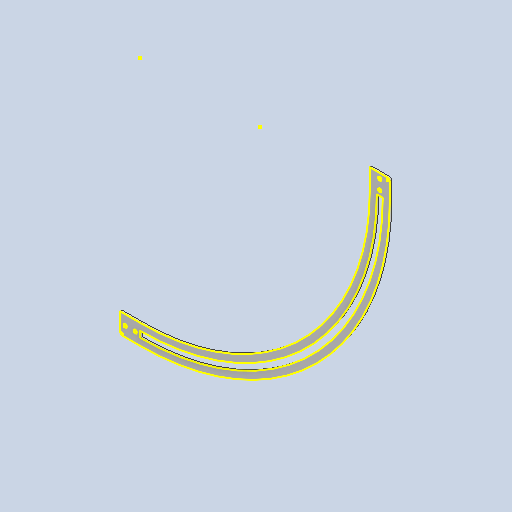
# Autodesk Inventor part: xx_memo
Saved by Autodesk Inventor 2025.1 (Build 291241000, 241)
## iProperties
Created: 2024-12-06
Part Number: xx_memo
Material: 一般
Document SubType Name: Modeling
Designer: yuki0520
Density: 1 g/cm^3
Appearance: 既定
Author: yuki0520
Autodesk Inventor part; units mm, degrees
ref_plane "YZ Plane" through (0, 0, 0) normal (1, 0, 0) x (0, 1, 0)
ref_plane "XZ Plane" through (0, 0, 0) normal (0, 1, 0) x (-1, 0, 0)
ref_plane "XY Plane" through (0, 0, 0) normal (0, 0, 1) x (1, 0, 0)
sketch "スケッチ1" plane through (0, 0, 0) normal (0, 0, 1) x (1, 0, 0)
  line L0 (120, -35) -> (-120, -35)
  line L1 (-120, -35) -> (-120, 35)
  line L2 (-120, 35) -> (120, 35)
  line L3 (120, 35) -> (120, -35)
  line L4 (120, -35) -> (-120, 35) construction
  line L5 (-120, -35) -> (120, 35) construction
  line L6 (-110, -35) -> (-130, -35)
  line L7 (-130, -35) -> (-130, 75)
  line L8 (-130, 75) -> (-110, 75)
  line L9 (-110, 75) -> (-110, -35)
  line L10 (110, 35) -> (130, 35)
  circle A0 centre (-120, 0) radius 6
  line L11 (110, 35) -> (130, 35)
  arc A1 (-120, -240) -> (120, 0) centre (-120, 0) ccw
  arc A2 (-120, -250) -> (130, 0) centre (-120, 0) ccw
  arc A3 (-120, -230) -> (110, 0) centre (-120, 0) ccw
  line L12 (110, 0) -> (130, 0)
  line L13 (130, 0) -> (130, 20)
  line L14 (130, 20) -> (110, 20)
  line L15 (110, 20) -> (110, 0)
  line L16 (-120, -250) -> (-140, -250)
  line L17 (-140, -250) -> (-140, -230)
  line L18 (-140, -230) -> (-120, -230)
  line L19 (-120, -230) -> (-120, -250)
  arc A4 (-120, -243) -> (123, 0) centre (-120, 0) ccw
  arc A5 (-120, -237) -> (117, 0) centre (-120, 0) ccw
  line L20 (130, 20) -> (-140, 20)
  line L21 (-140, 20) -> (-140, -250)
  line L22 (-140, -250) -> (130, -250)
  line L23 (130, -250) -> (130, 20)
  line L24 (-120, -250) -> (-120, 0)
  line L25 (-120, 0) -> (130, 0)
  point P0 (0, 0)
  point P1 (120, 25)
  point P2 (117, 0)
  point P3 (123, 0)
  point P4 (-120, -243)
  point P5 (-120, -237)
  dimension "d0" = 240
  dimension "d1" = 70
  dimension "d2" = 20
  dimension "d3" = 110
  dimension "d4" = 10
  dimension "d8" = 12
  dimension "d14" = 10
  dimension "d18" = 10
  dimension "d19" = 10
  dimension "d20" = 20
  dimension "d21" = 20
  dimension "d22" = 20
  dimension "d23" = 20
  dimension "d26" = 3
  dimension "d27" = 3
  dimension "d37" = 20
  constraints: 52 end point, 10 parallel, 10 point on circle, 7 horizontal, 6 centre point, 6 perpendicular, 4 midpoint, 3 point on line, 1 coincident, 1 other
  measures "d0" distance of L1.end L2.end
  measures "d1" distance of L0.end L1.end
  measures "d2" distance of L7.end L8.end
  measures "d3" distance of L6.end L7.end
  measures "d4" distance between parallel lines of L9 L1
  measures "d8" diameter of A0
  measures "d14" distance from line of L11 point (120, 25)
  measures "d18" radial gap between concentric circles of A1 A2
  measures "d19" radial gap between concentric circles of A1 A3
  measures "d20" distance of L14.end L13.end
  measures "d21" distance of L13.end L12.end
  measures "d22" distance of L18.end L17.end
  measures "d23" distance of L16.end L17.end
  measures "d26" radial gap between concentric circles of A1 A4
  measures "d27" radial gap between concentric circles of A1 A5
  measures "d37" distance between parallel lines of L21 L24
extrude "押し出し1" add sketch "スケッチ1" along normal blind 2 contours A3 L12 A5 L0 | L0 A5 L19 A3 | L19 L16 L17 L18 | L15 L14 L3 L12 | L3 L14 L13 L12 | L19 A4 L12 A2
sketch "スケッチ2" plane through (0, 0, 2) normal (0, 0, 1) x (1, 0, 0)
  line L0 (130, 20) -> (110, 20) projected
  line L1 (120, 20) -> (120, 0)
  line L2 (117, 0) -> (123, 0) projected
  line L3 (-140, -230) -> (-140, -250) projected
  line L4 (-140, -240) -> (-120, -240)
  point P0 (0, 0)
  point P1 (120, 15)
  point P2 (120, 5)
  point P3 (-135, -240)
  point P4 (-125, -240)
  dimension "d28" = 10
  dimension "d29" = 5
  dimension "d52" = 10
  dimension "d53" = 5
  constraints: 4 end point, 4 point on line, 3 midpoint, 1 horizontal
  measures "d28" distance of point (120, 15) point (120, 5)
  measures "d29" distance from line of L0 point (120, 15)
  measures "d52" distance of point (-135, -240) point (-125, -240)
  measures "d53" horizontal distance of L3.start point (-135, -240)
hole "穴1" at (120, 15, 2) at (120, 5, 2) at (-125, -240, 2) at (-135, -240, 2) direction (0, 0, -1) diameter 3.4 end through all
fillet "フィレット1" radius 2 2 edges at (130, 20, 1) (-140, -250, 1)
sketch "スケッチ5" plane through (0, 0, 2) normal (0, 0, 1) x (1, 0, 0)
  arc A0 (-140, -248) -> (-138, -250) centre (-138, -248) ccw projected
  line L0 (-138, -250) -> (-120, -250) projected
  arc A1 (-120, -250) -> (130, 0) centre (-120, 0) ccw projected
  line L1 (130, 0) -> (130, 18) projected
  arc A2 (130, 18) -> (128, 20) centre (128, 18) ccw projected
  line L2 (128, 20) -> (110, 20) projected
  line L3 (110, 20) -> (110, 0) projected
  arc A3 (-120, -230) -> (110, 0) centre (-120, 0) ccw projected
  line L4 (-120, -230) -> (-140, -230) projected
  line L5 (-140, -230) -> (-140, -248) projected
  circle A4 centre (-135, -240) radius 1.7 projected
  circle A5 centre (-125, -240) radius 1.7 projected
  circle A6 centre (120, 5) radius 1.7 projected
  circle A7 centre (120, 15) radius 1.7 projected
  line L6 (117, 0) -> (123, 0) projected
  arc A8 (-120, -243) -> (123, 0) centre (-120, 0) ccw projected
  line L7 (-120, -243) -> (-120, -237) projected
  arc A9 (-120, -237) -> (117, 0) centre (-120, 0) ccw projected
  point P0 (0, 0)
equation "\"d4\" = 0.5 * d2"
equation "\"d14\" = 0.5 * d10"
equation "\"d27\" = d26"
equation "\"d52\" = d28"
equation "\"d53\" = d29"
equation "\"d10\" = 20"
